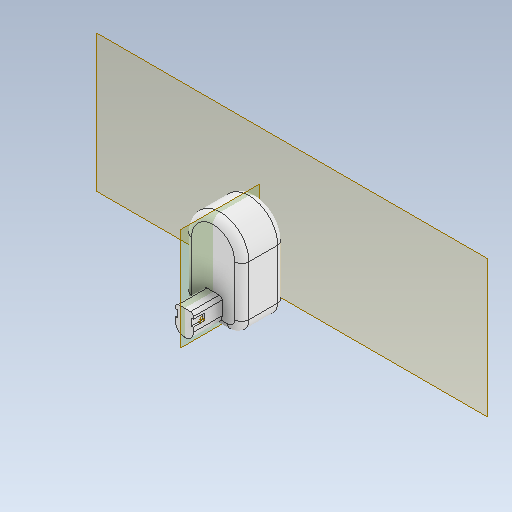
# Autodesk Inventor part: spacer_battery_pack
Saved by Autodesk Inventor 2020 (Build 240168000, 168)
## iProperties
Created: 2020-02-18
Part Number: spacer_battery_pack
Material: ABS Plastic
Document SubType Name: Modeling
Designer: erwin
Density: 1.06 g/cm^3
Appearance: Smooth - White
Mass: 624.151 g
Surface Area: 423.728 cm^2
Volume: 588.822 cm^3
Author: erwin
Autodesk Inventor part; units mm, degrees
ref_plane "YZ Plane" through (0, 0, 0) normal (1, 0, 0) x (0, 1, 0)
ref_plane "XZ Plane" through (0, 0, 0) normal (0, 1, 0) x (-1, 0, 0)
ref_plane "XY Plane" through (0, 0, 0) normal (0, 0, 1) x (1, 0, 0)
ref_plane "Work Plane1" through (0, 0, 0) normal (0, 0, 1) x (1, 0, 0)
sketch "Sketch1" plane through (0, 0, 0) normal (0, 0, 1) x (1, 0, 0)
  line L0 (-89.8092, 15.4671) -> (-9.8092, 15.4671)
  line L1 (-9.8092, 15.4671) -> (-9.8092, -114.5329)
  line L2 (-9.8092, -114.5329) -> (-89.8092, -114.5329)
  line L3 (-89.8092, -114.5329) -> (-89.8092, 15.4671)
  point P0 (0, 0)
  dimension "d0" = 80
  dimension "d1" = 130
  constraints: 8 end point, 2 parallel, 1 horizontal, 1 perpendicular
  measures "d0" distance of L1.end L2.end
  measures "d1" distance of L0.end L1.end
extrude "Extrusion1" add sketch "Sketch1" along normal blind 60
sketch "Sketch2" plane through (0, 0, 60) normal (0, 0, 1) x (1, 0, 0)
  line L0 (-62.3092, -75.5329) -> (-37.3092, -75.5329)
  line L1 (-37.3092, -75.5329) -> (-37.3092, -110.5329)
  line L2 (-37.3092, -110.5329) -> (-62.3092, -110.5329)
  line L3 (-62.3092, -110.5329) -> (-62.3092, -75.5329)
  line L4 (-89.8092, -114.5329) -> (-9.8092, -114.5329) projected
  line L5 (-9.8092, -114.5329) -> (-9.8092, 15.4671) projected
  line L6 (-89.8092, 15.4671) -> (-89.8092, -114.5329) projected
  point P0 (0, 0)
  dimension "d4" = 25
  dimension "d5" = 35
  dimension "d6" = 4
  dimension "d7" = 27.5
  dimension "d8" = 27.5
  constraints: 8 end point, 2 parallel, 1 horizontal, 1 perpendicular
  measures "d4" distance of L1.end L2.end
  measures "d5" distance of L0.end L1.end
  measures "d6" distance between parallel lines of L4 L2
  measures "d7" distance between parallel lines of L5 L1
  measures "d8" distance between parallel lines of L6 L3
extrude "Extrusion2" add sketch "Sketch2" along normal blind 40
fillet "Fillet1" radius 12 2 edges at (-62.3092, -110.5329, 80) (-37.3092, -110.5329, 80)
fillet "Fillet1" radius 4 2 edges at (-62.3092, -75.5329, 80) (-37.3092, -75.5329, 80)
fillet "Fillet2" radius 20 2 edges at (-89.8092, -114.5329, 30) (-9.8092, -114.5329, 30)
fillet "Fillet2" radius 40 2 edges at (-89.8092, 15.4671, 30) (-9.8092, 15.4671, 30)
fillet "Fillet3" radius 10 16 edges at (-83.9513, -108.675, 0) (-49.8092, -114.5329, 0) (-15.667, -108.675, 0) (-9.8092, -59.5329, 0) (-78.0935, 3.7514, 0) (-21.5249, 3.7514, 0) (-49.8092, 15.4671, 0) (-89.8092, -59.5329, 0) (-83.9513, -108.675, 60) (-49.8092, -114.5329, 60) (-15.667, -108.675, 60) (-9.8092, -59.5329, 60) (-78.0935, 3.7514, 60) (-21.5249, 3.7514, 60) (-49.8092, 15.4671, 60) (-89.8092, -59.5329, 60)
sketch "Sketch3" plane through (0, 0, 100) normal (0, 0, 1) x (1, 0, 0)
  line L0 (-62.3092, -98.5329) -> (-62.3092, -79.5329) projected
  line L1 (-62.3092, -82.8005) -> (-59.6618, -82.8005)
  line L2 (-59.6618, -82.8005) -> (-59.6618, -92.3283)
  line L3 (-59.6618, -92.3283) -> (-62.3092, -92.3283)
  line L4 (-62.3092, -92.3283) -> (-62.3092, -82.8005)
  point P0 (0, 0)
  constraints: 8 end point, 2 parallel, 1 horizontal, 1 perpendicular, 1 point on line
extrude "Extrusion3" cut sketch "Sketch3" against normal blind 15
ref_plane "Work Plane2" through (-49.8092, -98.5329, 60) normal (-1, 0, 0) x (0, 0, 1)
mirror "Mirror1" about plane through (-49.8092, -98.5329, 60) normal (-1, 0, 0) of "Extrusion3"
equation "\"d8\" = d7"
body "Solid1"
